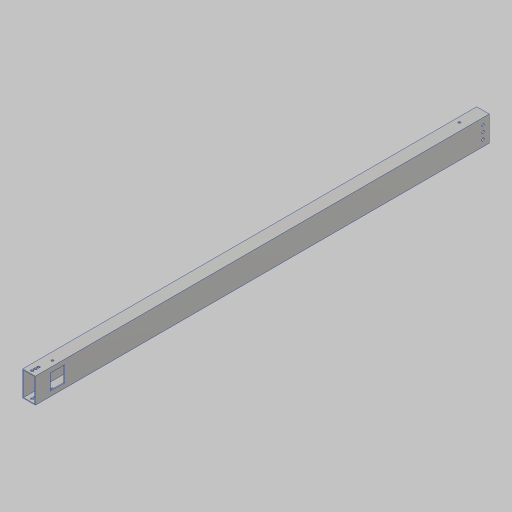
# Autodesk Inventor part: EL2-004
Saved by Autodesk Inventor 2023.5 (Build 275446000, 446)
## iProperties
RuleStatus: InUse
Created: 2025-01-11
Part Number: EL2-004
Material: Aluminum 6061
Document SubType Name: Modeling
Designer: mavericks
Mass: 304.185 g
Surface Area: 718.547 cm^2
Volume: 112.661 cm^3
Density: 2.7 g/cm^3
Appearance: Aluminum - Flat
AfterDocNew0: SHOW
AfterDocOpen0: SHOW
Author: mavericks
Autodesk Inventor part; units mm, degrees
ref_plane "YZ Plane" through (0, 0, 0) normal (1, 0, 0) x (0, 1, 0)
ref_plane "XZ Plane" through (0, 0, 0) normal (0, 1, 0) x (-1, 0, 0)
ref_plane "XY Plane" through (0, 0, 0) normal (0, 0, 1) x (1, 0, 0)
sketch "Sketch1" plane through (0, 0, 0) normal (0, 0, 1) x (1, 0, 0)
  line L0 (-12.7, -25.4) -> (12.7, -25.4)
  line L1 (12.7, -25.4) -> (12.7, 25.4)
  line L2 (12.7, 25.4) -> (-12.7, 25.4)
  line L3 (-12.7, 25.4) -> (-12.7, -25.4)
  line L4 (-12.7, -25.4) -> (12.7, 25.4) construction
  line L5 (12.7, -25.4) -> (-12.7, 25.4) construction
  line L6 (-11.1125, 23.8125) -> (11.1125, 23.8125)
  line L7 (11.1125, 23.8125) -> (11.1125, -23.8125)
  line L8 (11.1125, -23.8125) -> (-11.1125, -23.8125)
  line L9 (-11.1125, -23.8125) -> (-11.1125, 23.8125)
  point P0 (0, 0)
  dimension "width" = 25.4
  dimension "height" = 50.8
  dimension "thickness" = 1.5875
  constraints: 20 end point, 4 parallel, 2 midpoint, 2 perpendicular, 1 horizontal, 3 other
  measures "width" distance of L2.end L1.end
  measures "height" distance of L1.end L0.end
  measures "thickness" distance between parallel lines of L2 L6
extrude "Extrusion1" add sketch "Sketch1" along normal mid plane 914.4
sketch "Sketch2" plane through (-12.7, 25.4, 457.2) normal (0, 1, 0) x (1, 0, 0)
  line L0 (25.4, 0) -> (0, 0) projected
  line L1 (0, 914.4) -> (0, 0) projected
  point P0 (12.7, 457.2)
  point P1 (12.7, 6.35)
  point P2 (12.7, 12.7)
  point P3 (12.7, 19.05)
  point P4 (12.7, 0)
  point P5 (12.7, 0)
  dimension "d5" = 6.35
  dimension "d6" = 6.35
  dimension "d7" = 6.35
  constraints: 3 vertical alignment, 2 midpoint
  measures "d5" distance of point (12.7, 0) point (12.7, 6.35)
  measures "d6" distance of point (12.7, 12.7) point (12.7, 6.35)
  measures "d7" distance of point (12.7, 19.05) point (12.7, 12.7)
hole "Hole1" at (0, 25.4, 450.85) at (0, 25.4, 444.5) at (0, 25.4, 438.15) direction (0, -1, 0) diameter 5.1054 end through all clearance for "Flat Head Machine Screw (82)" size "#10" standard "Ansi Unified Screw Threads"
sketch "Sketch3" plane through (-12.7, -25.4, 457.2) normal (-1, 0, 0) x (0, 0, 1)
  line L0 (-914.4, 0) -> (-914.4, 50.8) projected
  point P0 (-457.2, 25.4)
  point P1 (-901.7, 38.1)
  point P2 (-901.7, 25.4)
  point P3 (-901.7, 12.7)
  point P4 (-914.4, 25.4)
  dimension "d15" = 12.7
  dimension "d16" = 12.7
  dimension "d17" = 12.7
  constraints: 2 vertical alignment, 1 horizontal alignment, 1 midpoint
  measures "d15" distance from line of L0 point (-901.7, 38.1)
  measures "d16" distance of point (-901.7, 25.4) point (-901.7, 38.1)
  measures "d17" distance of point (-901.7, 12.7) point (-901.7, 25.4)
hole "Hole2" at (-12.7, 12.7, -444.5) at (-12.7, 0, -444.5) at (-12.7, -12.7, -444.5) direction (1, 0, 0) diameter 5.1054 end through all clearance for "Flat Head Machine Screw (82)" size "#10" standard "Ansi Unified Screw Threads"
sketch "Sketch4" plane through (-12.7, 25.4, 457.2) normal (0, 1, 0) x (1, 0, 0)
  circle A0 centre (12.7, 19.05) radius 2.5527 projected
  line L0 (25.4, 914.4) -> (25.4, 0) projected
  point P0 (12.7, 457.2)
  point P1 (15.4686, 44.45)
  dimension "d34" = 9.9314
  dimension "d55" = 25.4
  measures "d34" distance from line of L0 point (15.469, 44.45)
  measures "d55" vertical distance of point (15.469, 44.45) A0.centre
hole "Hole3" at (2.7686, 25.4, 412.75) direction (0, -1, 0) diameter 4.445 end through all
sketch "Sketch5" plane through (-12.7, 25.4, 457.2) normal (0, 1, 0) x (1, 0, 0)
  line L0 (0, 914.4) -> (25.4, 914.4) projected
  line L1 (0, 914.4) -> (0, 0) projected
  point P0 (12.7, 457.2)
  point P1 (9.9314, 869.95)
  point P2 (12.7, 914.4)
  dimension "d35" = 44.45
  dimension "d36" = 9.9314
  constraints: 1 midpoint
  measures "d35" vertical distance of point (12.7, 914.4) point (9.931, 869.95)
  measures "d36" distance from line of L1 point (9.931, 869.95)
hole "Hole4" at (-2.7686, 25.4, -412.75) direction (0, -1, 0) diameter 4.445 end through all
sketch "Sketch6" plane through (12.7, -25.4, 457.2) normal (1, 0, 0) x (0, 0, -1)
  line L0 (58.42, 41.275) -> (30.48, 41.275)
  line L1 (30.48, 41.275) -> (30.48, 9.525)
  line L2 (30.48, 9.525) -> (58.42, 9.525)
  line L3 (58.42, 9.525) -> (58.42, 41.275)
  line L4 (58.42, 41.275) -> (30.48, 9.525) construction
  line L5 (30.48, 41.275) -> (58.42, 9.525) construction
  line L6 (0, 0) -> (0, 50.8) projected
  line L7 (914.4, 50.8) -> (0, 50.8) projected
  point P0 (457.2, 25.4)
  point P1 (44.45, 25.4)
  point P2 (0, 25.4)
  dimension "d44" = 30.48
  dimension "d45" = 27.94
  dimension "d47" = 31.75
  constraints: 12 end point, 3 midpoint, 2 parallel, 1 horizontal, 1 horizontal alignment, 1 perpendicular
  measures "d44" distance between parallel lines of L6 L1
  measures "d45" distance of L0.start L0.end
  measures "d47" distance between parallel lines of L2 L0
extrude "Extrusion2" cut sketch "Sketch6" against normal blind 1.5875
sketch "Sketch7" plane through (-12.7, -25.4, 457.2) normal (-1, 0, 0) x (0, 0, 1)
  line L0 (-883.92, 9.525) -> (-855.98, 9.525)
  line L1 (-855.98, 9.525) -> (-855.98, 41.275)
  line L2 (-855.98, 41.275) -> (-883.92, 41.275)
  line L3 (-883.92, 41.275) -> (-883.92, 9.525)
  line L4 (-883.92, 9.525) -> (-855.98, 41.275) construction
  line L5 (-855.98, 9.525) -> (-883.92, 41.275) construction
  line L6 (-914.4, 0) -> (-914.4, 50.8) projected
  point P0 (-457.2, 25.4)
  point P1 (-869.95, 25.4)
  point P2 (-914.4, 25.4)
  dimension "d50" = 30.48
  dimension "d51" = 31.75
  dimension "d52" = 27.94
  constraints: 12 end point, 3 midpoint, 2 parallel, 1 horizontal, 1 horizontal alignment, 1 perpendicular
  measures "d50" distance from line of point (-914.4, 25.4) L3
  measures "d51" distance between parallel lines of L2 L0
  measures "d52" distance between parallel lines of L3 L1
extrude "Extrusion3" cut sketch "Sketch7" against normal blind 1.5875
equation "\"d6\" = d5"
equation "\"d7\" = d6"
equation "\"d17\" = d16"
body "Solid1"
